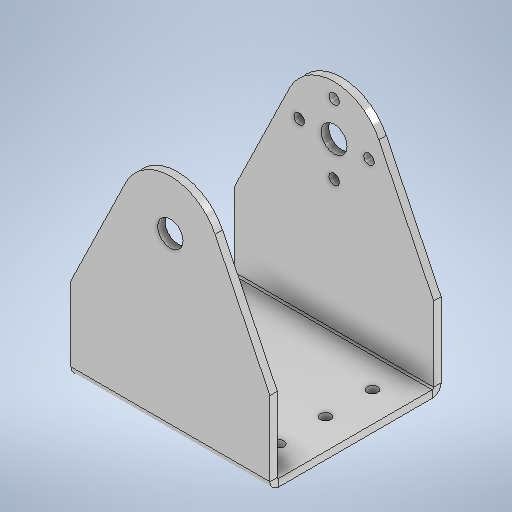
# Autodesk Inventor part: axis_12_bottom_frame(top)
Saved by Autodesk Inventor 2025.2 (Build 292293000, 293)
## iProperties
Created: 2025-05-04
Part Number: axis_12_bottom_frame(top)
Material: Aluminum 6061-AHC
Document SubType Name: Sheet Metal
Designer: User
Density: 2.7 g/cm^3
Sheet Metal Rule: Default_mm
Appearance: Aluminum - Dark
Flat Pattern Width: 4 cm
Flat Pattern Length: 11.8989 cm
Flat Pattern Area: 47.5954 cm^2
Sheet Metal Width: 40.000 mm
Sheet Metal Length: 118.989 mm
Sheet Metal Area: 4759.542 mm^2
Author: User
Autodesk Inventor part; units mm, degrees
ref_plane "YZ Plane" through (0, 0, 0) normal (1, 0, 0) x (0, 1, 0)
ref_plane "XZ Plane" through (0, 0, 0) normal (0, 1, 0) x (-1, 0, 0)
ref_plane "XY Plane" through (0, 0, 0) normal (0, 0, 1) x (1, 0, 0)
sketch "Sketch1" plane through (0, 0, 0) normal (0, 1, 0) x (-1, 0, 0)
  line L0 (20, -15.715) -> (-20, -15.715)
  line L1 (-20, -15.715) -> (-20, 15.715)
  line L2 (-20, 15.715) -> (20, 15.715)
  line L3 (20, 15.715) -> (20, -15.715)
  point P0 (0, 0)
  dimension "d0" = 40
  dimension "d1" = 20
  dimension "d2" = 31.43
  dimension "d3" = 15.715
  measures "d0" distance of L0.start L0.end
  measures "d1" distance from line of point (0, 0) L3
  measures "d2" distance of L0.end L1.end
  measures "d3" distance from line of point (0, 0) L0
extrude "Plate1" add sketch "Sketch1" along normal blind 1.5
sketch "Sketch2" plane through (20, 0, 17.215) normal (0, 0, -1) x (-1, 0, 0)
  line L0 (40, 0) -> (0, 0)
  line L1 (0, 0) -> (0, 45)
  line L2 (0, 45) -> (40, 45)
  line L3 (40, 45) -> (40, 0)
  constraints: 8 end point
edge flange "Flange1" height 45 angle 90 thickness 1.5 bend radius 0.31 thickness toward (0, 0, -1) relief tear relief width 1.5 relief depth 0.75 edges at (0, 1.5, 15.715) wall of the first edge with corners at (-20, 0, 17.215) (20, 0, 17.215) (20, 45, 17.215) (-20, 45, 17.215)
bend "Bend1"
corner "Corner1"
sketch "Sketch3" plane through (-20, 0, -17.215) normal (0, 0, 1) x (1, 0, 0)
  line L0 (40, 0) -> (0, 0)
  line L1 (0, 0) -> (0, 45)
  line L2 (0, 45) -> (40, 45)
  line L3 (40, 45) -> (40, 0)
  constraints: 8 end point
edge flange "Flange2" height 45 angle 90 thickness 1.5 bend radius 0.31 thickness toward (0, 0, 1) relief tear relief width 1.5 relief depth 0.75 edges at (0, 1.5, -15.715) wall of the first edge with corners at (20, 0, -17.215) (-20, 0, -17.215) (-20, 45, -17.215) (20, 45, -17.215)
bend "Bend2"
corner "Corner2"
sketch "Sketch4" plane through (-20, 45, 17.215) normal (0, 0, 1) x (1, 0, 0)
  line L0 (0, -43.19) -> (0, 0) projected
  line L1 (0, 0) -> (40, 0) projected
  line L2 (40, 0) -> (40, -43.19) projected
  line L3 (0, -43.19) -> (40, -43.19) projected
  arc A0 (28.9876, -5.6156) -> (11.0124, -5.6156) centre (20, -10) ccw
  line L4 (0, -38.19) -> (40, -38.19)
  line L5 (40, -38.19) -> (40, -28.19)
  line L6 (40, -28.19) -> (0, -28.19)
  line L7 (0, -28.19) -> (0, -38.19)
  line L8 (40, -28.19) -> (28.9876, -5.6156)
  line L9 (11.0124, -5.6156) -> (0, -28.19)
  point P0 (0, -28.19)
  point P1 (20, 0)
  point P2 (40, -28.19)
  dimension "d50" = 10
  dimension "d51" = 20
  dimension "d52" = 20
  dimension "d53" = 38.19
  dimension "d54" = 10
  dimension "d55" = 40
  dimension "d56" = 40
  constraints: 12 end point, 2 parallel, 2 point on circle, 2 tangent, 1 centre point, 1 horizontal, 1 perpendicular
  measures "d50" distance from line of L1 A0.centre
  measures "d51" diameter of A0
  measures "d52" distance from line of L0 A0.centre
  measures "d53" distance between parallel lines of L4 L1
  measures "d54" distance between parallel lines of L4 L6
  measures "d55" distance between parallel lines of L2 L7
  measures "d56" distance between parallel lines of L0 L5
extrude "Extrusion1" cut sketch "Sketch4" against normal blind 50 contours L0 L1 A0 L9 | L8 A0 L1 L2
sketch "Sketch6" plane through (-20, 1.81, 17.215) normal (0, 0, 1) x (1, 0, 0)
  arc A0 (28.9876, 37.5744) -> (11.0124, 37.5744) centre (20, 33.19) ccw projected
  point P0 (20, -1.81)
hole "Hole2" at (0, 35, 17.215) direction (0, 0, -1) diameter 5.1 depth 1.5 clearance for "Hex Head Bolt" size "M5" standard "Ansi Metric M Profile"
sketch "Sketch7" plane through (-20, 1.81, -15.715) normal (0, 0, 1) x (1, 0, 0)
  arc A0 (28.9876, 37.5744) -> (11.0124, 37.5744) centre (20, 33.19) ccw projected
  point P0 (20, -1.81)
hole "Hole3" at (0, 35, -15.715) direction (0, 0, -1) diameter 5.2 depth 1.5 clearance for "Hex Head Bolt" size "M5" standard "Ansi Metric M Profile"
sketch "Sketch8" plane through (0, 1.5, 0) normal (0, 1, 0) x (1, 0, 0)
  line L0 (20, 15.405) -> (20, -15.405) projected
  line L1 (20, -15.715) -> (-20, -15.715) projected
  line L2 (-20, -15.405) -> (20, -15.405) projected
  line L3 (20, 15.405) -> (-20, 15.405) projected
  point P0 (0, 0)
  point P1 (14, -9.405)
  point P2 (-14, -9.405)
  point P3 (14, 0)
  point P4 (-14, 0)
  point P5 (14, 9.405)
  point P6 (-14, 9.405)
  dimension "d71" = 6
  dimension "d73" = 6
  dimension "d76" = 28
  dimension "d79" = 9.405
  constraints: 1 horizontal, 1 vertical, 5 other
  measures "d71" distance from line of L0 point (14, -9.405)
  measures "d73" distance from line of point (14, -9.405) L2
  measures "d76" distance of point (14, -9.405) point (-14, -9.405)
  measures "d79" distance of point (14, -9.405) point (14, 0)
hole "Hole4" at (14, 1.5, 9.405) at (-14, 1.5, 9.405) at (14, 1.5, 0) at (-14, 1.5, 0) at (14, 1.5, -9.405) at (-14, 1.5, -9.405) direction (0, -1, 0) diameter 2.1 depth 1.5
sketch "Sketch9" plane through (20, 1.81, -17.215) normal (0, 0, -1) x (-1, 0, 0)
  arc A0 (28.9876, 37.5744) -> (11.0124, 37.5744) centre (20, 33.19) ccw projected
  circle A1 centre (20, 40.19) radius 1.05
  circle A2 centre (13, 33.19) radius 1.05
  circle A3 centre (20, 26.19) radius 1.05
  circle A4 centre (27, 33.19) radius 1.05
  point P0 (20, -1.81)
  dimension "d89" = 7
  dimension "d90" = 0
  dimension "d91" = 2.1
  dimension "d94" = 360
  constraints: 4 centre point, 9 other
  measures "d89" distance of A0.centre A1.centre
  measures "d90" horizontal distance of A0.centre A1.centre
  measures "d91" diameter of A1
hole "Hole5" at (0, 28, -17.215) at (7, 35, -17.215) at (-7, 35, -17.215) at (0, 42, -17.215) direction (0, 0, 1) diameter 2.1 depth 1.5
equation "\"d62\" = Thickness"
equation "\"d69\" = Thickness"
equation "\"d87\" = Thickness"
equation "\"d101\" = Thickness"
equation "\"d4\" = Thickness"
equation "\"d5\" = BendReliefWidth"
equation "\"d6\" = BendReliefDepth"
equation "\"d7\" = MinimumRemnant"
equation "\"d8\" = TransitionRadius"
equation "\"d11\" = BendRadius"
equation "\"d12\" = CornerReliefSize"
equation "\"d13\" = GapSize"
equation "\"d14\" = JacobiRadiusSize"
equation "\"d15\" = BendReliefWidth"
equation "\"d16\" = BendReliefDepth"
equation "\"d17\" = MinimumRemnant"
equation "\"d18\" = TransitionRadius"
equation "\"d21\" = BendRadius"
equation "\"d22\" = CornerReliefSize"
equation "\"d23\" = GapSize"
equation "\"d24\" = JacobiRadiusSize"
equation "\"BendReliefWidth\" = Thickness"
equation "\"BendReliefDepth\" = 0.5 * Thickness"
equation "\"CornerReliefSize\" = 4 * Thickness"
equation "\"MinimumRemnant\" = 2 * Thickness"
equation "\"TransitionRadius\" = BendRadius"
equation "\"JacobiRadiusSize\" = BendRadius"
equation "\"GapSize\" = Thickness"
equation "\"Thickness\" = 1.5"
equation "\"BendRadius\" = 0.31"
body "Solid1"
